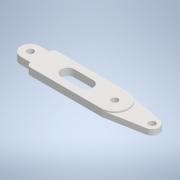
# Autodesk Inventor part: Pieza 5
Saved by Autodesk Inventor 2021 (Build 250183000, 183)
## iProperties
Created: 2021-03-31
Part Number: Pieza 5
Material: Generic
Document SubType Name: Modeling
Designer: trejo
Density: 1 g/cm^3
Appearance: Default
Author: trejo
Autodesk Inventor part; units mm, degrees
ref_plane "YZ Plane" through (0, 0, 0) normal (1, 0, 0) x (0, 1, 0)
ref_plane "XZ Plane" through (0, 0, 0) normal (0, 1, 0) x (-1, 0, 0)
ref_plane "XY Plane" through (0, 0, 0) normal (0, 0, 1) x (1, 0, 0)
sketch "Sketch1" plane through (0, 0, 0) normal (0, 1, 0) x (-1, 0, 0)
  line L0 (-5, 0) -> (5, 0) construction
  line L1 (-5, -3.5) -> (5, -3.5)
  line L2 (5, 3.5) -> (-5, 3.5)
  arc A0 (-5, 3.5) -> (-5, -3.5) centre (-5, 0) ccw
  arc A1 (5, -3.5) -> (5, 3.5) centre (5, 0) ccw
  circle A2 centre (-20, 0) radius 1.75
  arc A3 (-20, 7.4) -> (-20, -7.4) centre (-20, 0) ccw
  line L3 (17.5, -7.4) -> (-20, -7.4)
  line L4 (17.5, 7.4) -> (-20, 7.4)
  line L5 (20, 4.9) -> (20, -4.9)
  arc A4 (25, -5) -> (25, 5) centre (25, 0) ccw
  circle A5 centre (25, 0) radius 1.75
  line L6 (25, 5) -> (19.998, 5)
  line L7 (25, -5) -> (19.998, -5)
  arc A6 (20, 4.9) -> (17.5, 7.4) centre (17.5, 4.9) ccw
  arc A7 (17.5, -7.4) -> (20, -4.9) centre (17.5, -4.9) ccw
  circle A8 centre (-40, 0) radius 1.75
  circle A9 centre (-40, 0) radius 3.75
  line L8 (-40, 3.75) -> (-21.3747, 7.2712)
  line L9 (-40, -3.75) -> (-21.3747, -7.2712)
  point P0 (0, 0)
  dimension "d3" = 10
  dimension "d4" = 3.5
  dimension "d5" = 3.5
  dimension "d6" = 14.8
  dimension "d10" = 10
  dimension "d11" = 5
  dimension "d12" = 3.5
  dimension "d13" = 2.5
  dimension "d51" = 15
  dimension "d52" = 40
  dimension "d53" = 3.5
  dimension "d54" = 7.5
  dimension "d55" = 20
  constraints: 22 end point, 18 point on circle, 11 tangent, 10 centre point, 3 coincident, 2 parallel, 1 equal radius, 1 horizontal, 1 midpoint, 1 perpendicular, 1 vertical
  measures "d3" distance of L0.start L0.end
  measures "d4" radius of A0
  measures "d5" diameter of A2
  measures "d6" diameter of A3
  measures "d10" diameter of A4
  measures "d11" distance from line of L5 A4.centre
  measures "d12" diameter of A5
  measures "d13" radius of A6
  measures "d51" distance from line of L5 L0.end
  measures "d52" distance from line of L5 A2.centre
  measures "d53" diameter of A8
  measures "d54" diameter of A9
  measures "d55" distance of A2.centre A9.centre
extrude "Extrusion1" add sketch "Sketch1" along normal mid plane 3.8 contours L4 A6 L5 A7 L3 A3
sketch "Sketch4" plane through (0, 0, 0) normal (0, 1, 0) x (-1, 0, 0)
  line L0 (-5, 0) -> (5, 0) construction
  line L1 (-5, -3.5) -> (5, -3.5)
  line L2 (5, 3.5) -> (-5, 3.5)
  arc A0 (-5, 3.5) -> (-5, -3.5) centre (-5, 0) ccw
  arc A1 (5, -3.5) -> (5, 3.5) centre (5, 0) ccw
  circle A2 centre (-20, 0) radius 1.75
  arc A3 (-20, 7.4) -> (-20, -7.4) centre (-20, 0) ccw
  line L3 (17.5, -7.4) -> (-20, -7.4)
  line L4 (17.5, 7.4) -> (-20, 7.4)
  line L5 (20, 4.9) -> (20, -4.9)
  arc A4 (25, -5) -> (25, 5) centre (25, 0) ccw
  circle A5 centre (25, 0) radius 1.75
  line L6 (25, 5) -> (19.998, 5)
  line L7 (25, -5) -> (19.998, -5)
  arc A6 (20, 4.9) -> (17.5, 7.4) centre (17.5, 4.9) ccw
  arc A7 (17.5, -7.4) -> (20, -4.9) centre (17.5, -4.9) ccw
  circle A8 centre (-40, 0) radius 1.75
  arc A9 (-40.6844, 3.687) -> (-40.6844, -3.687) centre (-40, 0) ccw
  line L8 (-21.3505, 7.2757) -> (-40.6844, 3.687)
  arc A10 (-20, 7.4) -> (-20, -7.4) centre (-20, 0) ccw projected
  line L9 (-48.2908, 0) -> (-20.7624, 0) construction
  line L10 (-40.6844, -3.687) -> (-21.3505, -7.2757)
  point P0 (0, 0)
  point P1 (0, 0)
  dimension "d56" = 10
  dimension "d57" = 3.5
  dimension "d58" = 3.5
  dimension "d59" = 14.8
  dimension "d60" = 10
  dimension "d61" = 5
  dimension "d62" = 3.5
  dimension "d63" = 2.5
  dimension "d64" = 15
  dimension "d65" = 40
  dimension "d66" = 3.5
  dimension "d67" = 7.5
  dimension "d68" = 20
  constraints: 24 end point, 18 point on circle, 14 tangent, 10 centre point, 3 coincident, 2 horizontal, 2 parallel, 1 equal radius, 1 midpoint, 1 perpendicular, 1 vertical
  measures "d56" distance of L0.start L0.end
  measures "d57" radius of A0
  measures "d58" diameter of A2
  measures "d59" diameter of A3
  measures "d60" diameter of A4
  measures "d61" distance from line of L5 A4.centre
  measures "d62" diameter of A5
  measures "d63" radius of A6
  measures "d64" distance from line of L5 L0.end
  measures "d65" distance from line of L5 A2.centre
  measures "d66" diameter of A8
  measures "d67" diameter of A9
  measures "d68" distance of A2.centre A9.centre
extrude "Extrusion4" add sketch "Sketch4" along normal blind 1.1 and the other way blind 1.9 contours A3 L10 A9 L8
sketch "Sketch5" plane through (0, 0, 0) normal (0, 1, 0) x (-1, 0, 0)
  line L0 (-5, 0) -> (5, 0) construction
  line L1 (-5, -3.5) -> (5, -3.5)
  line L2 (5, 3.5) -> (-5, 3.5)
  arc A0 (-5, 3.5) -> (-5, -3.5) centre (-5, 0) ccw
  arc A1 (5, -3.5) -> (5, 3.5) centre (5, 0) ccw
  circle A2 centre (-20, 0) radius 1.75
  arc A3 (-20, 7.4) -> (-20, -7.4) centre (-20, 0) ccw
  line L3 (17.5, -7.4) -> (-20, -7.4)
  line L4 (17.5, 7.4) -> (-20, 7.4)
  line L5 (20, 4.9) -> (20, -4.9)
  arc A4 (25, -5) -> (25, 5) centre (25, 0) ccw
  circle A5 centre (25, 0) radius 1.75
  line L6 (25, 5) -> (19.998, 5)
  line L7 (25, -5) -> (19.998, -5)
  arc A6 (20, 4.9) -> (17.5, 7.4) centre (17.5, 4.9) ccw
  arc A7 (17.5, -7.4) -> (20, -4.9) centre (17.5, -4.9) ccw
  circle A8 centre (-40, 0) radius 1.75
  circle A9 centre (-40, 0) radius 3.75
  line L8 (-40, 3.75) -> (-21.3747, 7.2712)
  line L9 (-40, -3.75) -> (-21.3747, -7.2712)
  point P0 (0, 0)
  point P1 (0, 0)
  dimension "d73" = 10
  dimension "d74" = 3.5
  dimension "d75" = 3.5
  dimension "d76" = 14.8
  dimension "d77" = 10
  dimension "d78" = 5
  dimension "d79" = 3.5
  dimension "d80" = 2.5
  dimension "d81" = 15
  dimension "d82" = 40
  dimension "d83" = 3.5
  dimension "d84" = 7.5
  dimension "d85" = 20
  constraints: 22 end point, 18 point on circle, 11 tangent, 10 centre point, 3 coincident, 2 parallel, 1 equal radius, 1 horizontal, 1 midpoint, 1 perpendicular, 1 vertical
  measures "d73" distance of L0.start L0.end
  measures "d74" radius of A0
  measures "d75" diameter of A2
  measures "d76" diameter of A3
  measures "d77" diameter of A4
  measures "d78" distance from line of L5 A4.centre
  measures "d79" diameter of A5
  measures "d80" radius of A6
  measures "d81" distance from line of L5 L0.end
  measures "d82" distance from line of L5 A2.centre
  measures "d83" diameter of A8
  measures "d84" diameter of A9
  measures "d85" distance of A2.centre A9.centre
extrude "Extrusion5" add sketch "Sketch5" along normal blind 1.9 and the other way blind 0.8 contours L6 A4 L7 A7 L5 A6
move faces "Move1" translate (0, -0.1, 0) faces at (-21.0833, -0.8, 0)
body "Solid1"
